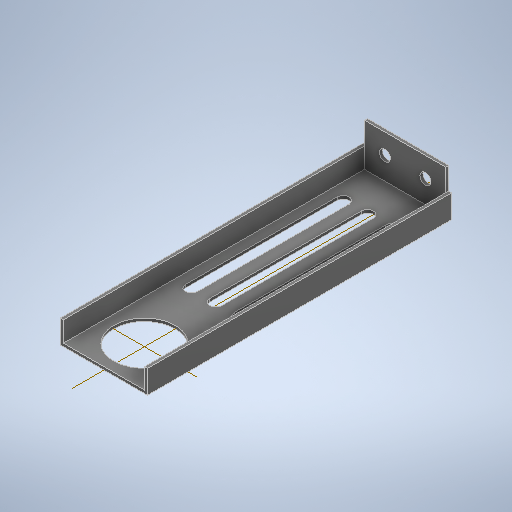
# Autodesk Inventor part: Support Frame (Filament Holder
Saved by Autodesk Inventor 2025 (Build 290162000, 162)
## iProperties
Manager: J. Wilburn
Created: 2025-03-12
Part Number: Support Frame (Filament Holder
Material: Steel, Wrought
Document SubType Name: Modeling
Designer: MAL16204
Density: 7.85 g/cm^3
Appearance: Smooth - Black
Mass: 95.2342 g
Surface Area: 177.701 cm^2
Volume: 12.1317 cm^3
Author: Richard Malstrom
Title: Support Frame (Filament Holder)
Subject: Ender 3 Pro Assembly
Autodesk Inventor part; units mm, degrees
ref_plane "YZ Plane" through (0, 0, 0) normal (1, 0, 0) x (0, 1, 0)
ref_plane "XZ Plane" through (0, 0, 0) normal (0, 1, 0) x (-1, 0, 0)
ref_plane "XY Plane" through (0, 0, 0) normal (0, 0, 1) x (1, 0, 0)
sketch "Sketch1" plane through (0, 0, 0) normal (0, 1, 0) x (-1, 0, 0)
  circle A0 centre (0, 0) radius 15.2
  line L0 (21.5, 20) -> (-21.5, 20)
  line L1 (-21.5, 20) -> (-21.5, -130)
  line L2 (-21.5, -130) -> (21.5, -130)
  line L3 (21.5, -130) -> (21.5, 20)
  line L4 (0, -160) -> (0, 50) projected
  line L5 (12, -35.2) -> (12, -110) construction
  line L6 (15, -35.2) -> (15, -110)
  line L7 (9, -110) -> (9, -35.2)
  arc A1 (15, -35.2) -> (9, -35.2) centre (12, -35.2) ccw
  arc A2 (9, -110) -> (15, -110) centre (12, -110) ccw
  line L8 (0, -35.2) -> (0, -110) construction
  line L9 (3, -35.2) -> (3, -110)
  line L10 (-3, -110) -> (-3, -35.2)
  arc A3 (3, -35.2) -> (-3, -35.2) centre (0, -35.2) ccw
  arc A4 (-3, -110) -> (3, -110) centre (0, -110) ccw
  line L11 (-12, -35.2) -> (-12, -110) construction
  line L12 (-9, -35.2) -> (-9, -110)
  line L13 (-15, -110) -> (-15, -35.2)
  arc A5 (-9, -35.2) -> (-15, -35.2) centre (-12, -35.2) ccw
  arc A6 (-15, -110) -> (-9, -110) centre (-12, -110) ccw
  line L14 (12, -72.6) -> (-12, -72.6) construction
  point P0 (0, 20)
  point P1 (0, -72.6)
  dimension "d0" = 30.4
  dimension "d1" = 43
  dimension "d2" = 150
  dimension "d3" = 20
  dimension "d4" = 74.8
  dimension "d5" = 6
  dimension "d6" = 20
  dimension "d7" = 74.8
  dimension "d8" = 6
  dimension "d9" = 74.8
  dimension "d10" = 6
  dimension "d11" = 24
  constraints: 28 end point, 12 point on circle, 7 centre point, 6 tangent, 6 vertical, 5 midpoint, 2 parallel, 2 perpendicular, 2 point on line, 1 coincident, 1 horizontal, 15 other
  measures "d0" diameter of A0
  measures "d1" distance between parallel lines of L3 L1
  measures "d2" distance between parallel lines of L2 L0
  measures "d3" distance from line of L0 point (0, 0)
  measures "d4" distance of L5.end L5.start
  measures "d6" distance from line of L2 L5.end
  measures "d7" distance of L8.end L8.start
  measures "d9" distance of L11.end L11.start
  measures "d11" distance of L14.end L14.start
extrude "Extrusion1" add sketch "Sketch1" along normal blind 1.5 contours A0 L4 L0 L3 L2 A4 L9 A3 | A0 L4 A3 L10 A4 L2 L1 L0
sketch "Sketch2" plane through (0, 1.5, 0) normal (0, 1, 0) x (1, 0, 0)
  line L0 (-21.5, 130) -> (-21.5, -20) projected
  line L1 (-21.5, -20) -> (-20, -20)
  line L2 (-20, -20) -> (-20, 130)
  line L3 (-20, 130) -> (-21.5, 130)
  line L4 (-21.5, 130) -> (-21.5, -20)
  line L5 (-21.5, -20) -> (21.5, -20) projected
  line L6 (21.5, 130) -> (-21.5, 130) projected
  line L7 (21.5, -20) -> (20, -20)
  line L8 (20, -20) -> (20, 130)
  line L9 (20, 130) -> (21.5, 130)
  line L10 (21.5, 130) -> (21.5, -20)
  point P0 (0, 0)
  dimension "d14" = 1.5
  dimension "d15" = 1.5
  constraints: 16 end point, 4 parallel, 2 horizontal, 2 perpendicular, 1 point on line
  measures "d14" distance of L0.start L2.end
  measures "d15" distance between parallel lines of L10 L8
extrude "Extrusion2" add sketch "Sketch2" along normal blind 10 contours L3 L2 L1 L0 | L6 L10 L5 L8
sketch "Sketch3" plane through (0, 1.5, 0) normal (0, 1, 0) x (1, 0, 0)
  line L0 (-20, 130) -> (-20, -20) projected
  line L1 (-20, 130) -> (20.1092, 130)
  line L2 (20.1092, 130) -> (20.1092, 128.5)
  line L3 (20.1092, 128.5) -> (-20, 128.5)
  line L4 (-20, 128.5) -> (-20, 130)
  point P0 (0, 0)
  point P1 (-20, 128.5)
  dimension "d18" = 1.5
  constraints: 8 end point, 2 parallel, 1 horizontal, 1 perpendicular
  measures "d18" distance between parallel lines of L1 L3
extrude "Extrusion3" add sketch "Sketch3" along normal blind 21
sketch "Sketch4" plane through (-20, 1.5, -128.5) normal (0, 0, 1) x (1, 0, 0)
  line L0 (40, 0) -> (0, 0) projected
  line L1 (0, 21) -> (40.1092, 21) construction
  point P0 (20, -1.5)
  point P1 (10.068, 11)
  point P2 (30.0412, 11)
  point P3 (20.0546, 11.517)
  point P4 (20.0546, 21)
  dimension "d21" = 11
  dimension "d23" = 10
  dimension "d24" = 10
  constraints: 1 horizontal alignment, 1 midpoint, 1 vertical alignment
  measures "d21" distance from line of L0 point (10.068, 11)
  measures "d23" distance of point (20.055, 11.517) point (10.068, 11)
  measures "d24" distance of point (30.041, 11) point (20.055, 11.517)
hole "Hole1" at (-9.932, 12.5, -128.5) at (10.0412, 12.5, -128.5) direction (0, 0, -1) diameter 5.43 end through all
body "Solid1"
